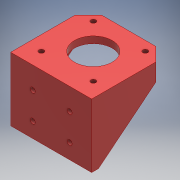
# Autodesk Inventor part: Ucwyt_NEMA17
Saved by Autodesk Inventor 2017 (Build 210142000, 142)
## iProperties
Created: 2018-08-10
Part Number: Ucwyt_NEMA17
Material: Ogólny
Document SubType Name: Modeling
Designer: Wojciech
Density: 1 g/cm^3
Appearance: Gładki - czerwony
Author: Wojciech
Autodesk Inventor part; units mm, degrees
ref_plane "YZ Plane" through (0, 0, 0) normal (1, 0, 0) x (0, 1, 0)
ref_plane "XZ Plane" through (0, 0, 0) normal (0, 1, 0) x (-1, 0, 0)
ref_plane "XY Plane" through (0, 0, 0) normal (0, 0, 1) x (1, 0, 0)
sketch "Szkic5" plane through (0, 0, 0) normal (1, 0, 0) x (0, 1, 0)
  line L0 (0, 0) -> (4, 0)
  line L1 (4, 0) -> (4, -38)
  line L2 (4, -38) -> (0, -38)
  line L3 (0, -38) -> (0, 0)
  line L4 (4, 0) -> (46.3, 0)
  line L5 (46.3, 0) -> (46.3, -4)
  line L6 (46.3, -4) -> (4, -4)
  line L7 (4, -4) -> (4, 0)
  dimension "d10" = 4
  dimension "d11" = 38
  dimension "d12" = 42.3
  dimension "d13" = 4
  constraints: 16 end point, 4 parallel, 2 horizontal, 2 perpendicular
  measures "d10" distance of L1.end L2.end
  measures "d11" distance of L0.end L1.end
  measures "d12" distance of L5.end L6.end
  measures "d13" distance of L4.end L5.end
extrude "Wyciągnięcie proste2" add sketch "Szkic5" along normal blind 48.3
sketch "Szkic6" plane through (0, 4, -4) normal (0, 1, 0) x (1, 0, 0)
  line L0 (48.3, -4) -> (48.3, 34) projected
  line L1 (48.3, 34) -> (45.3, 34)
  line L2 (45.3, 34) -> (45.3, 0)
  line L3 (45.3, 0) -> (48.3, 0)
  line L4 (48.3, 0) -> (48.3, 34)
  line L5 (0, -4) -> (0, 34) projected
  line L6 (0, 34) -> (3, 34)
  line L7 (3, 34) -> (3, 0)
  line L8 (3, 0) -> (0, 0)
  line L9 (0, 0) -> (0, 34)
  dimension "d16" = 3
  dimension "d17" = 34
  dimension "d18" = 3
  dimension "d19" = 34
  constraints: 16 end point, 4 parallel, 2 horizontal, 2 perpendicular
  measures "d16" distance of L3.end L2.end
  measures "d17" distance of L2.end L1.end
  measures "d18" distance of L7.end L8.end
  measures "d19" distance of L6.end L7.end
extrude "Wyciągnięcie proste3" add sketch "Szkic6" along normal blind 42.3
sketch "Szkic7" plane through (0, 0, 0) normal (-1, 0, 0) x (0, 0, 1)
  line L0 (-4, 46.3) -> (-38, 46.3) projected
  line L1 (-4, 46.3) -> (-38, 46.3)
  line L2 (-38, 4) -> (-38, 46.3) projected
  line L3 (-38, 46.3) -> (-38, 4)
  line L4 (-38, 4) -> (-4, 46.3)
  point P0 (0, 0)
  constraints: 6 end point, 2 collinear
extrude "Wyciągnięcie proste4" cut sketch "Szkic7" against normal through all
sketch "Szkic8" plane through (45.3, 4, -4) normal (0, 0, -1) x (-1, 0, 0)
  line L0 (45.3, 42.3) -> (-3, 42.3) projected
  line L1 (-3, 0) -> (-3, 42.3) projected
  line L2 (0, 42.3) -> (0, 0) projected
  circle A0 centre (21.15, 21.15) radius 11.25
  point P0 (45.3, -4)
  dimension "d24" = 21.15
  dimension "d26" = 21.15
  dimension "d27" = 22.5
  constraints: 1 centre point, 1 coincident
  measures "d24" distance from line of L0 point (21.15, 21.15)
  measures "d26" distance from line of point (21.15, 21.15) L2
  measures "d27" diameter of A0
extrude "Wyciągnięcie proste5" cut sketch "Szkic8" against normal blind 42.3
sketch "Szkic9" plane through (45.3, 4, -4) normal (0, 0, -1) x (-1, 0, 0)
  line L0 (45.3, 42.3) -> (-3, 42.3) projected
  line L1 (21.15, 42.3) -> (21.15, 0) construction
  line L2 (42.3, 0) -> (0, 0) projected
  line L3 (0, 42.3) -> (0, 0) projected
  line L4 (0, 21.15) -> (42.3, 21.15) construction
  line L5 (45.3, 42.3) -> (45.3, -4) projected
  point P0 (5.65, 36.65)
  point P1 (36.65, 36.65)
  point P2 (5.65, 5.65)
  point P3 (36.65, 5.65)
  dimension "d30" = 15.5
  dimension "d31" = 15.5
  constraints: 4 end point, 3 midpoint, 3 symmetric about line, 1 perpendicular
  measures "d30" distance from line of L1 point (5.65, 36.65)
  measures "d31" distance from line of L4 point (5.65, 36.65)
hole "Otwór1" at (39.65, 40.65, -4) at (8.65, 40.65, -4) at (39.65, 9.65, -4) at (8.65, 9.65, -4) direction (0, 0, 1) diameter 3 depth 8 tip angle 118
sketch "Szkic10" plane through (3, 4, -4) normal (0, 1, 0) x (1, 0, 0)
  line L0 (9.9, 0) -> (32.4, 0) projected
  line L1 (21.15, 0) -> (21.15, 34) construction
  line L2 (0, 34) -> (42.3, 34) projected
  line L3 (42.3, 0) -> (42.3, 34) projected
  line L4 (42.3, 17) -> (0, 17) construction
  line L5 (0, 34) -> (0, 0) projected
  point P0 (-3, -4)
  point P1 (32.15, 9)
  point P2 (10.15, 9)
  point P3 (32.15, 25)
  point P4 (10.15, 25)
  dimension "d39" = 11
  dimension "d40" = 8
  constraints: 4 end point, 4 midpoint, 3 symmetric about line
  measures "d39" distance from line of point (32.15, 9) L1
  measures "d40" distance from line of L4 point (32.15, 9)
hole "Otwór2" at (35.15, 4, -13) at (13.15, 4, -13) at (35.15, 4, -29) at (13.15, 4, -29) direction (0, -1, 0) diameter 3 depth 8 tip angle 118
chamfer "Faza1" distance 2 angle 45 4 edges at (35.15, 4, -14.5) (13.15, 4, -14.5) (35.15, 4, -30.5) (13.15, 4, -30.5)
chamfer "Faza2" distance 8 angle 45 2 edges at (48.3, 46.3, -2) (0, 46.3, -2)
